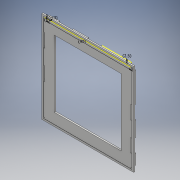
# Autodesk Inventor part: Slide_Final
Saved by Autodesk Inventor 2017 (Build 210142000, 142)
## iProperties
Created: 2018-11-05
Part Number: Slide_Final
Material: Generic
Document SubType Name: Modeling
Designer: Ralph
Density: 1 g/cm^3
Appearance: Default
Author: Ralph
Autodesk Inventor part; units mm, degrees
ref_plane "YZ Plane" through (0, 0, 0) normal (1, 0, 0) x (0, 1, 0)
ref_plane "XZ Plane" through (0, 0, 0) normal (0, 1, 0) x (-1, 0, 0)
ref_plane "XY Plane" through (0, 0, 0) normal (0, 0, 1) x (1, 0, 0)
sketch "Sketch1" plane through (0, 0, 0) normal (0, 1, 0) x (-1, 0, 0)
  line L0 (0, 0) -> (0, -90)
  line L1 (0, -90) -> (90, -90)
  line L2 (90, -90) -> (90, 0)
  line L3 (90, 0) -> (0, 0)
  line L4 (90, -90) -> (90, 0)
  line L5 (90, -90) -> (0, -90)
  line L6 (0, -90) -> (0, -91)
  line L7 (0, -91) -> (90, -91)
  line L8 (90, -91) -> (90, -90)
  line L9 (0, -90) -> (-1, -90)
  line L10 (-1, -90) -> (-1, 0)
  line L11 (-1, 0) -> (0, 0)
  line L12 (0, 0) -> (0, -90)
  line L13 (90, 0) -> (0, 0)
  line L14 (0, 0) -> (0, 1)
  line L15 (0, 1) -> (90, 1)
  line L16 (90, 1) -> (90, 0)
  line L17 (0, 0) -> (0, -10)
  line L18 (0, -10) -> (10, -10)
  line L19 (10, -10) -> (80, -10)
  line L20 (80, -10) -> (80, -80)
  line L21 (80, -80) -> (10, -80)
  line L22 (10, -80) -> (10, -10)
  line L23 (90, 0) -> (91, 0)
  line L24 (91, 0) -> (91, -90)
  line L25 (91, -90) -> (90, -90)
  line L26 (90, -90) -> (90, 0)
  dimension "d0" = 90
  dimension "d1" = 90
  dimension "d2" = 90
  dimension "d15" = 90
  dimension "d16" = 1
  dimension "d17" = 1
  dimension "d18" = 90
  dimension "d19" = 90
  dimension "d20" = 1
  dimension "d31" = 10
  dimension "d32" = 10
  dimension "d33" = 70
  dimension "d34" = 70
  dimension "d37" = 1
  dimension "d38" = 90
  constraints: 54 end point, 10 parallel, 9 perpendicular, 5 horizontal, 1 point on line, 1 vertical
  measures "d0" distance of L0.start L0.end
  measures "d1" distance of L0.end L1.end
  measures "d2" angle of L1 L0
  measures "d15" distance of L7.end L6.end
  measures "d16" distance of L6.end L5.end
  measures "d17" distance of L10.end L11.end
  measures "d18" distance of L9.end L10.end
  measures "d19" distance of L14.end L15.end
  measures "d20" distance of L13.end L14.end
  measures "d31" distance of L13.end L17.end
  measures "d32" distance of L17.end L18.end
  measures "d33" distance of L20.end L21.end
  measures "d34" distance of L19.end L20.end
  measures "d37" distance of L24.end L25.end
  measures "d38" distance of L23.end L24.end
extrude "Extrusion4" add sketch "Sketch1" along normal blind 1.5
sketch "Sketch5" plane through (0, 1.5, 0) normal (0, 1, 0) x (1, 0, 0)
  line L0 (0, -1) -> (0, 0) projected
  line L1 (-90, -1) -> (0, -1) projected
  line L2 (0, 0) -> (-90, 0)
  line L3 (-90, 0) -> (-90, -1)
  line L4 (-90, -1) -> (0, -1)
  line L5 (0, -1) -> (0, 0)
  line L6 (-90, 90) -> (-91, 90) projected
  line L7 (-90, 0) -> (-91, 0)
  line L8 (-91, 0) -> (-91, 90)
  line L9 (-91, 90) -> (-90, 90)
  line L10 (-90, 90) -> (-90, 0)
  line L11 (0, 90) -> (0, 91) projected
  line L12 (-90, 90) -> (0, 90)
  line L13 (0, 90) -> (0, 91)
  line L14 (0, 91) -> (-90, 91)
  line L15 (-90, 91) -> (-90, 90)
  line L16 (1, 0) -> (1, 90) projected
  line L17 (0, 90) -> (1, 90)
  line L18 (1, 90) -> (1, 0)
  line L19 (1, 0) -> (0, 0)
  line L20 (0, 0) -> (0, 90)
  dimension "d85" = 90
  dimension "d86" = 1
  constraints: 32 end point, 8 parallel, 4 horizontal, 4 perpendicular
  measures "d85" distance of L0.end L2.end
  measures "d86" distance of L2.end L1.start
extrude "Extrusion5" add sketch "Sketch5" along normal blind 1.5 contours L1 L3 L2 L0 | L20 L17 L16 L19 | L7 L8 L6 L10 | L12 L15 L14 L11
sketch "Sketch6" plane through (-90, 0, 1) normal (0, 0, 1) x (1, 0, 0)
  line L0 (90, 0) -> (90, 3) projected
  line L1 (90, 3) -> (88, 3)
  line L2 (90, 3) -> (0, 3) projected
  line L3 (88, 3) -> (57, 3)
  line L4 (57, 3) -> (57, 1.5)
  line L5 (57, 1.5) -> (88, 1.5)
  line L6 (88, 1.5) -> (88, 3)
  line L7 (57, 3) -> (43, 3)
  line L8 (43, 3) -> (27, 3)
  line L9 (27, 3) -> (27, 1.5)
  line L10 (27, 1.5) -> (43, 1.5)
  line L11 (43, 1.5) -> (43, 3)
  line L12 (27, 3) -> (13, 3)
  line L13 (13, 3) -> (2, 3)
  line L14 (2, 3) -> (2, 1.5)
  line L15 (2, 1.5) -> (13, 1.5)
  line L16 (13, 1.5) -> (13, 3)
  line L17 (2, 3) -> (0, 3)
  dimension "d41" = 2
  dimension "d42" = 31
  dimension "d43" = 1.5
  dimension "d44" = 14
  dimension "d45" = 16
  dimension "d46" = 1.5
  dimension "d47" = 14
  dimension "d48" = 11
  dimension "d49" = 1.5
  constraints: 32 end point, 6 parallel, 4 horizontal, 3 perpendicular, 3 point on line
  measures "d41" distance of L0.end L1.end
  measures "d42" distance of L5.end L4.end
  measures "d43" distance of L4.end L3.end
  measures "d44" distance of L3.end L7.end
  measures "d45" distance of L10.end L9.end
  measures "d46" distance of L9.end L8.end
  measures "d47" distance of L8.end L12.end
  measures "d48" distance of L15.end L14.end
  measures "d49" distance of L14.end L13.end
extrude "Extrusion6" add sketch "Sketch6" along normal blind 1.5
sketch "Sketch9" plane through (0, 0, -91) normal (0, 0, -1) x (-1, 0, 0)
  line L0 (90, 0) -> (90, 3)
  line L1 (90, 3) -> (88, 3)
  line L2 (90, 3) -> (0, 3)
  line L3 (88, 3) -> (57, 3)
  line L4 (57, 3) -> (57, 1.5)
  line L5 (57, 1.5) -> (88, 1.5)
  line L6 (88, 1.5) -> (88, 3)
  line L7 (57, 3) -> (43, 3)
  line L8 (43, 3) -> (27, 3)
  line L9 (27, 3) -> (27, 1.5)
  line L10 (27, 1.5) -> (43, 1.5)
  line L11 (43, 1.5) -> (43, 3)
  line L12 (27, 3) -> (13, 3)
  line L13 (13, 3) -> (2, 3)
  line L14 (2, 3) -> (2, 1.5)
  line L15 (2, 1.5) -> (13, 1.5)
  line L16 (13, 1.5) -> (13, 3)
  line L17 (2, 3) -> (0, 3)
  point P0 (0, 0)
  dimension "d52" = 2
  dimension "d53" = 31
  dimension "d54" = 1.5
  dimension "d55" = 14
  dimension "d56" = 16
  dimension "d57" = 1.5
  dimension "d58" = 14
  dimension "d59" = 11
  dimension "d60" = 1.5
  constraints: 36 end point, 6 parallel, 4 horizontal, 3 perpendicular, 3 point on line
  measures "d52" distance of L0.end L1.end
  measures "d53" distance of L5.end L4.end
  measures "d54" distance of L4.end L3.end
  measures "d55" distance of L3.end L7.end
  measures "d56" distance of L10.end L9.end
  measures "d57" distance of L9.end L8.end
  measures "d58" distance of L8.end L12.end
  measures "d59" distance of L15.end L14.end
  measures "d60" distance of L14.end L13.end
extrude "Extrusion7" add sketch "Sketch9" along normal blind 1.5
sketch "Sketch7" plane through (-91, 0, -90) normal (-1, 0, 0) x (0, 0, 1)
  line L0 (90, 1.5) -> (90, 3) projected
  line L1 (90, 3) -> (88, 3)
  line L2 (90, 3) -> (0, 3) projected
  line L3 (88, 3) -> (77, 3)
  line L4 (77, 3) -> (77, 1.5)
  line L5 (77, 1.5) -> (88, 1.5)
  line L6 (88, 1.5) -> (88, 3)
  line L7 (77, 3) -> (63, 3)
  line L8 (63, 3) -> (47, 3)
  line L9 (47, 3) -> (47, 1.5)
  line L10 (47, 1.5) -> (63, 1.5)
  line L11 (63, 1.5) -> (63, 3)
  line L12 (47, 3) -> (33, 3)
  line L13 (33, 3) -> (2, 3)
  line L14 (2, 3) -> (2, 1.5)
  line L15 (2, 1.5) -> (33, 1.5)
  line L16 (33, 1.5) -> (33, 3)
  line L17 (0, 0) -> (0, 3) projected
  line L18 (2, 3) -> (0, 3)
  point P0 (90, 0)
  dimension "d63" = 2
  dimension "d64" = 11
  dimension "d65" = 1.5
  dimension "d66" = 14
  dimension "d67" = 16
  dimension "d68" = 1.5
  dimension "d69" = 14
  dimension "d70" = 31
  dimension "d71" = 1.5
  constraints: 32 end point, 6 parallel, 4 horizontal, 3 perpendicular, 3 point on line
  measures "d63" distance of L0.end L1.end
  measures "d64" distance of L5.end L4.end
  measures "d65" distance of L4.end L3.end
  measures "d66" distance of L3.end L7.end
  measures "d67" distance of L10.end L9.end
  measures "d68" distance of L9.end L8.end
  measures "d69" distance of L8.end L12.end
  measures "d70" distance of L15.end L14.end
  measures "d71" distance of L14.end L13.end
extrude "Extrusion8" add sketch "Sketch7" along normal blind 1.5
sketch "Sketch8" plane through (1, 0, 0) normal (1, 0, 0) x (0, 0, -1)
  line L0 (90, 1.5) -> (90, 3)
  line L1 (90, 3) -> (88, 3)
  line L2 (90, 3) -> (0, 3)
  line L3 (88, 3) -> (77, 3)
  line L4 (77, 3) -> (77, 1.5)
  line L5 (77, 1.5) -> (88, 1.5)
  line L6 (88, 1.5) -> (88, 3)
  line L7 (77, 3) -> (63, 3)
  line L8 (63, 3) -> (47, 3)
  line L9 (47, 3) -> (47, 1.5)
  line L10 (47, 1.5) -> (63, 1.5)
  line L11 (63, 1.5) -> (63, 3)
  line L12 (47, 3) -> (33, 3)
  line L13 (33, 3) -> (2, 3)
  line L14 (2, 3) -> (2, 1.5)
  line L15 (2, 1.5) -> (33, 1.5)
  line L16 (33, 1.5) -> (33, 3)
  line L17 (0, 0) -> (0, 3)
  line L18 (2, 3) -> (0, 3)
  point P0 (0, 0)
  point P1 (90, 0)
  dimension "d74" = 2
  dimension "d75" = 11
  dimension "d76" = 1.5
  dimension "d77" = 14
  dimension "d78" = 16
  dimension "d79" = 1.5
  dimension "d80" = 14
  dimension "d81" = 31
  dimension "d82" = 1.5
  constraints: 38 end point, 6 parallel, 4 horizontal, 3 perpendicular, 3 point on line
  measures "d74" distance of L0.end L1.end
  measures "d75" distance of L5.end L4.end
  measures "d76" distance of L4.end L3.end
  measures "d77" distance of L3.end L7.end
  measures "d78" distance of L10.end L9.end
  measures "d79" distance of L9.end L8.end
  measures "d80" distance of L8.end L12.end
  measures "d81" distance of L15.end L14.end
  measures "d82" distance of L14.end L13.end
extrude "Extrusion9" add sketch "Sketch8" along normal blind 1.5
sketch "Sketch11" plane through (-90, 0, 1) normal (0, 0, 1) x (1, 0, 0)
  line L0 (0, 0) -> (90, 0) projected
  line L1 (0, 3) -> (2, 3) projected
  dimension "d87" = 3
  measures "d87" distance between parallel lines of L0 L1
sketch "Sketch12" plane through (0, 3, 0) normal (0, 1, 0) x (1, 0, 0)
  line L0 (-2, -2.5) -> (-33, -2.5) projected
  line L1 (0, 0) -> (-90, 0) projected
  dimension "d88" = 2.5
  measures "d88" distance between parallel lines of L0 L1
sketch "Sketch13" plane through (-91, 0, -90) normal (-1, 0, 0) x (0, 0, 1)
  line L0 (77, 1.5) -> (77, 3) projected
  line L1 (77, 3) -> (63, 3)
  line L2 (63, 3) -> (63, 0)
  line L3 (63, 0) -> (77, 0)
  line L4 (77, 0) -> (77, 3)
  line L5 (47, 1.5) -> (47, 3) projected
  line L6 (47, 3) -> (33, 3)
  line L7 (33, 3) -> (33, 0)
  line L8 (33, 0) -> (47, 0)
  line L9 (47, 0) -> (47, 3)
  point P0 (90, 0)
  dimension "d89" = 14
  dimension "d90" = 3
  dimension "d91" = 14
  dimension "d92" = 3
  constraints: 16 end point, 4 parallel, 2 horizontal, 2 perpendicular
  measures "d89" distance of L3.end L2.end
  measures "d90" distance of L2.end L1.end
  measures "d91" distance of L8.end L7.end
  measures "d92" distance of L7.end L6.end
extrude "Extrusion10" cut sketch "Sketch13" against normal blind 1.25
sketch "Sketch14" plane through (1, 0, 0) normal (1, 0, 0) x (0, 0, -1)
  line L0 (33, 3) -> (47, 3)
  line L1 (47, 3) -> (47, 0)
  line L2 (47, 0) -> (33, 0)
  line L3 (33, 0) -> (33, 3)
  line L4 (77, 3) -> (63, 3)
  line L5 (63, 3) -> (63, 0)
  line L6 (63, 0) -> (77, 0)
  line L7 (77, 0) -> (77, 3)
  point P0 (0, 0)
  dimension "d95" = 14
  dimension "d96" = 3
  dimension "d97" = 14
  dimension "d98" = 3
  constraints: 16 end point, 4 parallel, 2 horizontal, 2 perpendicular
  measures "d95" distance of L1.end L2.end
  measures "d96" distance of L0.end L1.end
  measures "d97" distance of L6.end L5.end
  measures "d98" distance of L5.end L4.end
extrude "Extrusion11" cut sketch "Sketch14" against normal blind 1.25
sketch "Sketch15" plane through (0, 0, 0) normal (0, -1, 0) x (1, 0, 0)
  line L0 (-90, -90) -> (-91, -90) projected
  line L1 (-91, -90) -> (-91.25, -90)
  line L2 (-91, -90) -> (-90.75, -90) construction
  line L3 (-91.25, -90) -> (-91.25, -91.25)
  line L4 (-91.25, -91.25) -> (1.25, -91.25)
  line L5 (1.25, -91.25) -> (1.25, 1.25)
  line L6 (1.25, 1.25) -> (-91.25, 1.25)
  line L7 (-91.25, 1.25) -> (-91.25, -91.25)
  line L8 (-93, -93) -> (3, -93)
  line L9 (3, -93) -> (3, 3)
  line L10 (3, 3) -> (-93, 3)
  line L11 (-93, 3) -> (-93, -93)
  line L12 (-91.25, -91.25) -> (-91.25, -93)
  line L13 (-91.25, -91.25) -> (-93, -91.25)
  point P0 (0, 0)
  dimension "d101" = 0.25
  dimension "d102" = 180
  dimension "d103" = 1.25
  dimension "d104" = 92.5
  dimension "d105" = 92.5
  dimension "d106" = 96
  dimension "d107" = 96
  dimension "d108" = 1.75
  dimension "d109" = 1.75
  constraints: 26 end point, 4 horizontal, 4 parallel, 4 perpendicular, 3 point on line, 1 collinear
  measures "d101" distance of L0.end L1.end
  measures "d102" angle of L1 L2
  measures "d103" distance of L1.end L3.end
  measures "d104" distance of L6.end L5.end
  measures "d105" distance of L5.end L4.end
  measures "d106" distance of L10.end L9.end
  measures "d107" distance of L9.end L8.end
  measures "d108" distance between parallel lines of L11 L12
  measures "d109" distance between parallel lines of L8 L13
extrude "Extrusion12" add sketch "Sketch15" against normal blind 1.3
body "Solid2"
